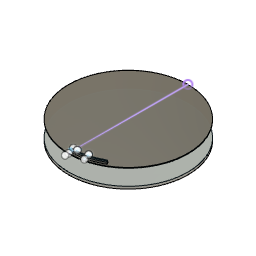
Table Furniture Design & LED holder v9 (Autodesk Fusion 360 design; units mm, degrees)
Autodesk Fusion 360 part; units mm, degrees
sketch "Sketch1" plane through (0, 0, 0) normal (0, 1, 0) x (1, 0, 0) in component "base"
  circle A0 centre (0, 0) radius 457.2
  dimension "d1" = 914.4
  constraint coincident A0.centre origin
  measures "d1" diameter of A0
extrude "Extrude1" add sketch "Sketch1" along normal blind 19.05 contours A0 picked at (169.517664, 35.545195) makes body 1 in component "base"
sketch "Sketch2" plane through (0, 19.05, 0) normal (0, 1, 0) x (-1, 0, 0) in component "base"
  circle A0 centre (0, 0) radius 457.2
sketch "Sketch1 (2)" plane through (0, 19.05, 0) normal (0, 1, 0) x (-1, 0, 0) in component "sand base"
sketch "Sketch2 (2)" plane through (0, 19.05, 0) normal (0, 1, 0) x (-1, 0, 0) in component "sand base"
  circle A0 centre (0, 0) radius 457.2
  constraint coincident A0.centre origin
extrude "Extrude1'" add sketch "Sketch2 (2)" along normal blind 5 separate body contours A0 picked at (169.517664, 35.545195) makes body 2 in component "sand base"
move_body "Move1" bodies 2 to x (1, 0, 0) y (0, 1, 0) z (0, 0, 1) at (0, 120, 0) in component "sand base"
sketch "Sketch1 (3)" plane through (0, 144.05, 0) normal (0, 1, 0) x (-1, 0, 0) in component "bezel"
  circle A0 centre (0, 0) radius 457.2
  circle A1 centre (0, 0) radius 457.2
  circle A2 centre (0, 0) radius 381
  dimension "d6" = 76.2
  constraint concentric A0 A1
  constraint concentric A1 A2
  measures "d6" distance of A1 A2
extrude "Extrude1''" add sketch "Sketch1 (3)" along normal blind 5 separate body contours A0 A1 picked at (430.097818, -22.714041) makes body 3 in component "bezel"
move_body "Move1'" bodies 3 to x (1, 0, 0) y (0, 1, 0) z (0, 0, 1) at (0, 30, 0) in component "bezel"
sketch "Sketch1 (4)" plane through (0, 179.05, 0) normal (0, 1, 0) x (-1, 0, 0) in component "glass"
  circle A0 centre (0, 0) radius 381
  circle A1 centre (0, 0) radius 457.2
  circle A2 centre (0, 0) radius 457.2
  constraint coincident A0.centre A1.centre
extrude "Extrude1'''" add sketch "Sketch1 (4)" along normal blind 6.35 separate body contours A0 | A1 A2 picked at (93.097588, 86.381938) picked at (430.097818, -22.714041) makes body 4 in component "glass"
sketch "Sketch1 (5)" plane through (0, 0, 0) normal (1, 0, 0) x (0, 0, -1) in component "skin"
sketch "Sketch2 (3)" plane through (0, 0, 0) normal (0, 0, 1) x (1, 0, 0) in component "skin"
  line L0 (472.2, 0) -> (457.2, 0)
  line L1 (457.2, 0) -> (457.2, 185.4)
  line L2 (457.2, 185.4) -> (472.2, 185.4)
  line L3 (472.2, 185.4) -> (472.2, 0)
  point P0 (457.2, 185.4)
  dimension "d11" = 15
  constraint horizontal L0
  constraint vertical L1
  constraint horizontal L2
  constraint vertical L3
  constraint coincident P0 L1.end
  measures "d11" distance of L1 L3
revolve "Revolve1" add sketch "Sketch2 (3)" angle 360 about axis through (0, 1.75, 0) along (0, 1, 0) separate body contours L0 L1 L2 L3 picked at (467.2, 61.8) makes body 5 in component "skin"
sketch "Sketch3" plane through (0, 0, 0) normal (0, 1, 0) x (1, 0, 0) in component "skin"
  line L0 (0, 474.000007) -> (0, 468.000007)
  line L1 (0, 468.000007) -> (1.500456, 468.000007)
  line L2 (0, 455.000007) -> (0, 461.370063)
  line L3 (0, 461.370063) -> (1.500456, 461.370063)
  arc A0 (1.500456, 461.370063) -> (1.500456, 468.000007) centre (1.500456, 464.685035) ccw
  constraint vertical L0
  constraint perpendicular L0 L1
  constraint vertical L2
  constraint perpendicular L2 L3
  constraint tangent L1 A0
  constraint tangent L3 A0
surface "Extrude1''''" add extruded along (0, 1, 0) between 0 and 195 path "Sketch3" along L2 L3 A0 L1 L0 separate body makes body 6 in component "skin"
thicken "Thicken1" add thickness 0.15 on both sides surfaces 6 separate body makes body 7 in component "skin"
pattern_circular "C-Pattern1" count 20 over 360 about axis through (0, 1.75, 0) along (0, 1, 0) of bodies 7 makes body 8 at (-138.765605, 130, -443.058062) makes body 9 at (-269.747259, 130, -374.121819) makes body 10 at (-377.754362, 130, -276.522762) makes body 11 at (-440.825399, 130, -148.42554) makes body 12 at (-462.030712, 130, -3.727697) makes body 13 at (-443.058062, 130, 138.765605) makes body 14 at (-374.121819, 130, 269.747259) makes body 15 at (-276.654555, 130, 377.64265) makes body 16 at (-148.453843, 130, 440.995833) makes body 17 at (-4.938538, 130, 464.254187) makes body 18 at (138.765605, 130, 443.058062) makes body 19 at (269.747259, 130, 374.121819) makes body 20 at (377.64265, 130, 276.654555) makes body 21 at (440.825399, 130, 148.42554) makes body 22 at (464.254187, 130, 4.938538) makes body 23 at (443.058062, 130, -138.765605) makes body 24 at (374.121819, 65, -269.747259) makes body 25 at (276.654555, 130, -377.64265) makes body 26 at (148.453843, 130, -440.995833) in component "skin"
combine "Combine1" operation cut target body 5 tool bodies 25 24 23 makes body 27 at (443.68294, 61.8, -161.611538) makes body 28 at (372.026839, 123.6, -290.807274) in component "skin"
sketch "Sketch1 (6)" plane through (0, 0, 0) normal (1, 0, 0) x (0, 0, -1) in component "LED Holder"
  line L0 (457.2, 144.05) -> (-457.2, 144.05)
  line L1 (-432.194301, 144.05) -> (-422.194301, 144.05)
  line L2 (-432.194301, 144.05) -> (-442.194301, 144.05)
  line L3 (-442.194301, 144.05) -> (-442.194301, 169.05)
  line L4 (-442.194301, 169.05) -> (-437.194301, 169.05)
  line L5 (-437.194301, 169.05) -> (-437.194301, 159.05)
  line L6 (-422.194301, 144.05) -> (-422.194301, 146.05)
  arc A0 (-437.194301, 159.05) -> (-422.194301, 146.05) centre (-421.901364, 161.54185) ccw
  line L7 (-442.194301, 169.05) -> (-450.194301, 169.05)
  arc A1 (-442.194301, 144.05) -> (-450.194301, 169.05) centre (-485.256801, 144.05) ccw
  dimension "d19" = 10
  dimension "d29" = 25
  dimension "d30" = 5
  dimension "d31" = 10
  dimension "d32" = 2
  dimension "d33" = 8
  constraint parallel L0 L1
  constraint perpendicular L0 L3
  constraint perpendicular L3 L4
  constraint perpendicular L4 L5
  constraint perpendicular L1 L6
  constraint perpendicular L3 L7
  constraint tangent L3 A1
revolve "Revolve2" add sketch "Sketch1 (6)" angle 30 about axis through (0, 1.75, 0) along (0, 1, 0) separate body contours L0 L1 L2 L3 L4 L5 L6 A0 | L3 L7 A1 picked at (-435.987566, 146.48404) picked at (-446.587497, 167.541977) makes body 29 in component "LED Holder"
sketch "Sketch4" plane through (0, 169.05, 0) normal (0, 1, 0) x (-1, 0, 0) in component "LED Holder"
  line L0 (0, 437.194301) -> (0, 450.194301)
  arc A0 (0, 450.194301) -> (-225.097151, 389.879702) centre (0, 0) ccw
  line L1 (-225.097151, 389.879702) -> (-218.597151, 378.621371)
  arc A1 (0, 437.194301) -> (-218.597151, 378.621371) centre (0, 0) ccw
  circle A2 centre (-111.205447, 415.572479) radius 7
  line L2 (-113.154212, 422.297267) -> (-124.58058, 462.075241)
  line L3 (-118.183814, 415.022568) -> (-117.000002, 400.000006)
  line L4 (-104.875611, 418.561322) -> (-98.000001, 404.000006)
  line L5 (-98.000001, 404.000006) -> (-117.000002, 400.000006)
  circle A3 centre (-111.205447, 415.572479) radius 2.5
  line L6 (-30.531279, 430.436382) -> (-26, 414.000006)
  circle A4 centre (-37.279532, 428.575983) radius 7
  line L7 (-44.243668, 429.283666) -> (-46.000001, 412.000006)
  line L8 (-26, 414.000006) -> (-46.000001, 412.000006)
  circle A5 centre (-37.279532, 428.575983) radius 2.5
  dimension "d35" = 14
  dimension "d36" = 5
  dimension "d41" = 14
  dimension "d42" = 5
  constraint tangent A1 A2
  constraint tangent A2 L3
  constraint tangent A2 L4
  constraint concentric A2 A3
  constraint tangent A4 L7
  constraint tangent L6 A4
  constraint tangent A1 A4
  constraint concentric A4 A5
  measures "d35" diameter of A2
  measures "d36" diameter of A3
  measures "d41" diameter of A4
  measures "d42" diameter of A5
extrude "Extrude5" cut sketch "Sketch4" against normal blind 28 contours A5 picked at (-37.464966, 429.388423) bodies 29 in component "LED Holder"
extrude "Extrude4" cut sketch "Sketch4" against normal blind 23 contours A2 | A2 L3 L4 L5 picked at (-106.066042, 417.490769) picked at (-108.139576, 404.268119) bodies 29 in component "LED Holder"
extrude "Extrude3" cut sketch "Sketch4" against normal blind 35 contours A3 picked at (-110.900996, 414.796751) bodies 29 in component "LED Holder"
extrude "Extrude6" cut sketch "Sketch4" against normal blind 23 contours A4 | L6 A4 L7 L8 picked at (-42.765095, 428.704273) picked at (-36.201072, 415.869581) bodies 29 in component "LED Holder"
sketch "Sketch5" plane through (0, 0, 0) normal (0, 1, 0) x (1, 0, 0) in component "LED Holder"
  circle A0 centre (0, 0) radius 445.4525
  circle A1 centre (0, 0) radius 457.2
  dimension "d47" = 890.905
  dimension "d48" = 914.4
  constraint coincident A0.centre A1.centre
  constraint concentric A0 A1
  measures "d47" diameter of A0
  measures "d48" diameter of A1
extrude "Extrude7" cut sketch "Sketch5" along normal blind 225 contours A1 picked at (449.923539, -44.844458) bodies 29 in component "LED Holder"
revolve "Revolve1'" [suppressed] in component "LED Holder"
sketch "Sketch2 (4)" plane through (0, 144.05, 0) normal (0, -1, 0) x (1, 0, 0) in component "LED Holder"
  line L0 (0, 442.194301) -> (0, 422.194301)
  arc A0 (178.427022, 382.637983) -> (0, 422.194301) centre (0, 0) ccw
  line L1 (178.427022, 382.637983) -> (186.879387, 400.764139)
  arc A1 (186.879387, 400.764139) -> (0, 442.194301) centre (0, 0) ccw
  circle A2 centre (95, 420) radius 2.5
  dimension "d23" = 5
  measures "d23" diameter of A2
extrude "Extrude1'''''" [suppressed] in component "LED Holder"
sketch "Sketch3 (2)" plane through (0, 164.05, 0) normal (0, 1, 0) x (-1, 0, 0) in component "LED Holder"
  circle A0 centre (-95, 420) radius 2.5
  line L0 (0, 422.194301) -> (0, 437.194301)
  arc A1 (0, 437.194301) -> (-184.766296, 396.2326) centre (0, 0) ccw
  line L1 (-184.766296, 396.2326) -> (-178.427022, 382.637983)
  arc A2 (0, 422.194301) -> (-178.427022, 382.637983) centre (0, 0) ccw
  circle A3 centre (-95, 420) radius 6.5
  line L2 (-101.012489, 417.530186) -> (-106.115385, 429.952625)
  line L3 (-88.5, 420) -> (-88.5, 435.594549)
  line L4 (-88.5, 435.594549) -> (-106.115385, 429.952625)
  dimension "d26" = 13
  constraint concentric A0 A3
  constraint tangent A3 L2
  constraint coincident A3 L3.start
  constraint tangent A3 L3
  constraint vertical L3
  measures "d26" diameter of A3
extrude "Extrude2" [suppressed] in component "LED Holder"
component "base" placed x (1, 0, 0) y (0, 1, 0) z (0, 0, 1) at (0, 0, 0)
component "sand base" placed x (1, 0, 0) y (0, 1, 0) z (0, 0, 1) at (0, 0, 0)
component "bezel" placed x (1, 0, 0) y (0, 1, 0) z (0, 0, 1) at (0, 0, 0)
component "glass" placed x (1, 0, 0) y (0, 1, 0) z (0, 0, 1) at (0, 0, 0)
component "skin" placed x (1, 0, 0) y (0, 1, 0) z (0, 0, 1) at (0, 0, 0)
component "LED Holder" placed x (1, 0, 0) y (0, 1, 0) z (0, 0, 1) at (0, 0, 0)
hidden bodies 6
equation "d1 = 36\""
equation "d6 = 3\""
equation "d48 = 36\""
